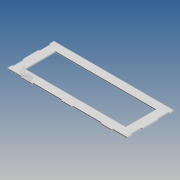
# Autodesk Inventor part: Carosserie_Capot_Avant_Haut
Saved by Autodesk Inventor 2019 (Build 230136000, 136)
## iProperties
Created: 2019-08-27
Part Number: Carosserie_Capot_Avant_Haut
Material: PVC-U
Document SubType Name: Modeling
Designer: jeremias.salamin
Density: 1.4 g/cm^3
Appearance: Lisse - Blanc
Description: Carosserie_Capot_Avant_haut
Author: jeremias.salamin
Autodesk Inventor part; units mm, degrees
ref_plane "YZ Plane" through (0, 0, 0) normal (1, 0, 0) x (0, 1, 0)
ref_plane "XZ Plane" through (0, 0, 0) normal (0, 1, 0) x (-1, 0, 0)
ref_plane "XY Plane" through (0, 0, 0) normal (0, 0, 1) x (1, 0, 0)
sketch "Sketch1" plane through (0, 0, 0) normal (0, 0, 1) x (1, 0, 0)
  line L0 (0, 24.5) -> (0, -24.5) construction
  line L1 (-63, 0) -> (63, 0) construction
  line L2 (45, -17.5) -> (-45, -17.5)
  line L3 (-45, -17.5) -> (-45, 17.5)
  line L4 (-45, 17.5) -> (45, 17.5)
  line L5 (45, 17.5) -> (45, -17.5)
  line L6 (45, -17.5) -> (-45, 17.5) construction
  line L7 (-45, -17.5) -> (45, 17.5) construction
  point P0 (0, 0)
  dimension "d0" = 90
  dimension "d1" = 35
  constraints: 12 end point, 2 midpoint, 2 parallel, 1 horizontal, 1 perpendicular
  measures "d0" distance of L3.end L4.end
  measures "d1" distance of L2.end L3.end
extrude "Extrusion1" add sketch "Sketch1" along normal mid plane 0.8
sketch "Esquisse2" plane through (0, 0, 0.4) normal (0, 0, 1) x (1, 0, 0)
  line L0 (-38, 11.5) -> (38, 11.5)
  line L1 (38, 11.5) -> (38, -11.5)
  line L2 (38, -11.5) -> (-38, -11.5)
  line L3 (-38, -11.5) -> (-38, 11.5)
  line L4 (-45, -17.5) -> (45, -17.5) construction
  line L5 (45, -17.5) -> (45, 17.5) construction
  line L6 (45, 17.5) -> (-45, 17.5) construction
  line L7 (-45, 17.5) -> (-45, -17.5) construction
  line L8 (0, 24.5) -> (0, -24.5) construction
  line L9 (-63, 0) -> (63, 0) construction
  point P0 (0, 0)
  dimension "d4" = 76
  dimension "d5" = 23
  constraints: 8 end point, 2 parallel, 1 horizontal, 1 perpendicular, 2 other
  measures "d4" distance of L1.end L2.end
  measures "d5" distance of L0.end L1.end
extrude "Extrusion2" cut sketch "Esquisse2" against normal blind 10
sketch "Esquisse4" plane through (0, 0, -0.4) normal (0, 0, -1) x (-1, 0, 0)
  line L0 (-45, 14.0096) -> (-44.2, 14.0096)
  line L1 (-44.2, 14.0096) -> (-44.2, 6.0096)
  line L2 (-44.2, 6.0096) -> (-45, 6.0096)
  line L3 (-45, 6.0096) -> (-45, 14.0096)
  line L4 (-44.2, -13.9904) -> (-45, -13.9904)
  line L5 (-45, -13.9904) -> (-45, -5.9904)
  line L6 (-45, -5.9904) -> (-44.2, -5.9904)
  line L7 (-44.2, -5.9904) -> (-44.2, -13.9904)
  line L8 (45, -13.9904) -> (44.2, -13.9904)
  line L9 (44.2, -13.9904) -> (44.2, -5.9904)
  line L10 (44.2, -5.9904) -> (45, -5.9904)
  line L11 (45, -5.9904) -> (45, -13.9904)
  line L12 (44.2, 14.0096) -> (45, 14.0096)
  line L13 (45, 14.0096) -> (45, 6.0096)
  line L14 (45, 6.0096) -> (44.2, 6.0096)
  line L15 (44.2, 6.0096) -> (44.2, 14.0096)
  point P0 (0, 0)
  constraints: 32 end point, 8 horizontal, 8 vertical, 16 other
extrude "Extrusion4" cut sketch "Esquisse4" against normal blind 0.8
sketch "Esquisse5" plane through (0, 0, 0.4) normal (0, 0, 1) x (1, 0, 0)
  line L0 (-44.2, 14.0096) -> (-45, 14.0096) construction
  line L1 (-45, 14.0096) -> (-45, 17.5) construction
  line L2 (-45, 17.5) -> (45, 17.5) construction
  line L3 (45, 17.5) -> (45, 14.0096) construction
  line L4 (45, 14.0096) -> (44.2, 14.0096) construction
  line L5 (44.2, 14.0096) -> (44.2, 6.0096) construction
  line L6 (44.2, 6.0096) -> (45, 6.0096) construction
  line L7 (45, 6.0096) -> (45, -5.9904) construction
  line L8 (45, -5.9904) -> (44.2, -5.9904) construction
  line L9 (44.2, -5.9904) -> (44.2, -13.9904) construction
  line L10 (44.2, -13.9904) -> (45, -13.9904) construction
  line L11 (45, -13.9904) -> (45, -17.5) construction
  line L12 (45, -17.5) -> (-45, -17.5) construction
  line L13 (-45, -17.5) -> (-45, -13.9904) construction
  line L14 (-45, -13.9904) -> (-44.2, -13.9904) construction
  line L15 (-44.2, -13.9904) -> (-44.2, -5.9904) construction
  line L16 (-44.2, -5.9904) -> (-45, -5.9904) construction
  line L17 (-45, -5.9904) -> (-45, 6.0096) construction
  line L18 (-45, 6.0096) -> (-44.2, 6.0096) construction
  line L19 (-44.2, 6.0096) -> (-44.2, 14.0096) construction
  line L20 (38, -11.5) -> (38, 11.5) construction
  line L21 (38, 11.5) -> (-38, 11.5) construction
  line L22 (-38, 11.5) -> (-38, -11.5) construction
  line L23 (-38, -11.5) -> (38, -11.5) construction
  line L24 (-38, -11.5) -> (-38, 11.5) construction
  line L25 (-38, 11.5) -> (38, 11.5) construction
  line L26 (38, 11.5) -> (38, -11.5) construction
  line L27 (38, -11.5) -> (-38, -11.5) construction
  line L28 (-45, -5.9904) -> (-44.2, -5.9904) construction
  line L29 (-44.2, -5.9904) -> (-44.2, -13.9904) construction
  line L30 (-44.2, -13.9904) -> (-45, -13.9904) construction
  line L31 (-45, -13.9904) -> (-45, -17.5) construction
  line L32 (-45, -17.5) -> (45, -17.5) construction
  line L33 (45, -17.5) -> (45, -13.9904) construction
  line L34 (45, -13.9904) -> (44.2, -13.9904) construction
  line L35 (44.2, -13.9904) -> (44.2, -5.9904) construction
  line L36 (44.2, -5.9904) -> (45, -5.9904) construction
  line L37 (45, -5.9904) -> (45, 6.0096) construction
  line L38 (45, 6.0096) -> (44.2, 6.0096) construction
  line L39 (44.2, 6.0096) -> (44.2, 14.0096) construction
  line L40 (44.2, 14.0096) -> (45, 14.0096) construction
  line L41 (45, 14.0096) -> (45, 17.5) construction
  line L42 (45, 17.5) -> (-45, 17.5) construction
  line L43 (-45, 17.5) -> (-45, 14.0096) construction
  line L44 (-45, 14.0096) -> (-44.2, 14.0096) construction
  line L45 (-44.2, 14.0096) -> (-44.2, 6.0096) construction
  line L46 (-44.2, 6.0096) -> (-45, 6.0096) construction
  line L47 (-45, 6.0096) -> (-45, -5.9904) construction
  line L48 (-63, 0) -> (63, 0) construction
  line L49 (0, 24.66) -> (0, -25.46) construction
  line L50 (-34, -17.5) -> (-26, -17.5)
  line L51 (-26, -17.5) -> (-26, -18.3)
  line L52 (-26, -18.3) -> (-34, -18.3)
  line L53 (-34, -18.3) -> (-34, -17.5)
  line L54 (-4, -18.3) -> (-4, -17.5)
  line L55 (-4, -17.5) -> (4, -17.5)
  line L56 (4, -17.5) -> (4, -18.3)
  line L57 (4, -18.3) -> (-4, -18.3)
  line L58 (26, -18.3) -> (26, -17.5)
  line L59 (26, -17.5) -> (34, -17.5)
  line L60 (34, -17.5) -> (34, -18.3)
  line L61 (34, -18.3) -> (26, -18.3)
  point P0 (0, 0)
  dimension "d32" = 8
  dimension "d33" = 0.8
  dimension "d36" = 30
  constraints: 24 end point, 2 horizontal, 2 parallel, 1 perpendicular, 1 point on line, 17 other
  measures "d32" distance of L51.end L52.end
  measures "d33" distance of L50.end L51.end
  measures "d36" distance of L52.end L54.start
extrude "Extrusion5" add sketch "Esquisse5" against normal blind 0.8
